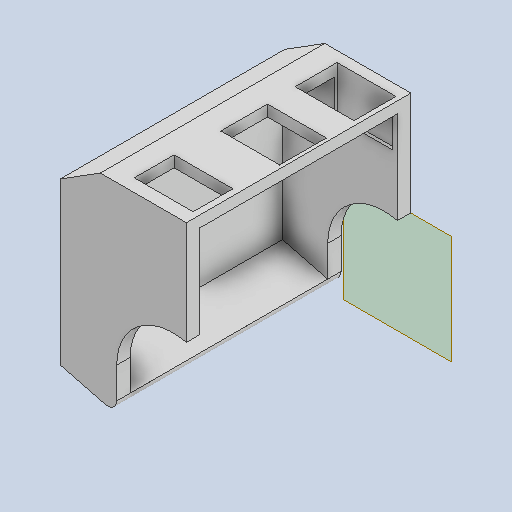
# Autodesk Inventor part: obudowa
Saved by Autodesk Inventor 2022 (Build 260153000, 153)
## iProperties
Created: 2022-12-13
Part Number: obudowa
Material: Generic
Document SubType Name: Modeling
Designer: komputer
Density: 1 g/cm^3
Appearance: Default
Author: komputer
Autodesk Inventor part; units mm, degrees
ref_plane "YZ Plane" through (0, 0, 0) normal (1, 0, 0) x (0, 1, 0)
ref_plane "XZ Plane" through (0, 0, 0) normal (0, 1, 0) x (-1, 0, 0)
ref_plane "XY Plane" through (0, 0, 0) normal (0, 0, 1) x (1, 0, 0)
sketch "Sketch1" plane through (0, 0, 0) normal (0, 0, 1) x (1, 0, 0)
  circle A0 centre (0, 0) radius 11 projected
  line L0 (9.8023, 37.5977) -> (3, 35.24) projected
  line L1 (3, 35.24) -> (3, 11.34) projected
  line L2 (3, 11.34) -> (9, 11.34) projected
  line L3 (9, 11.34) -> (9, 30.1331) projected
  line L4 (9, 30.1331) -> (7.9327, 24.5668) projected
  line L5 (7.9327, 24.5668) -> (7.3445, 24.6796) projected
  line L6 (7.3445, 24.6796) -> (9.8023, 37.5977) projected
  circle A1 centre (0, 0) radius 12.5167
  line L7 (-21, 24.5198) -> (-21, -3.96) projected
  line L8 (-19, -3.96) -> (-21, -3.96) projected
  line L9 (-19, 24.5198) -> (-19, -3.96) projected
  line L10 (-21, 24.5198) -> (-19, 24.5198) projected
  line L11 (-21, 28.5732) -> (-21, 24.5198) projected
  line L12 (-21, 24.5198) -> (-19, 24.5198) projected
  line L13 (-19, 28.5732) -> (-19, 24.5198) projected
  line L14 (-21, 28.5732) -> (-19, 28.5732) projected
  line L15 (1.6453, 33.2633) -> (-11.4547, 33.2633) projected
  line L16 (-19, 0.49) -> (-19, -3.96) projected
  line L17 (-14, 0.49) -> (-19, 0.49) projected
  line L18 (-14, -0.96) -> (-14, 0.49) projected
  arc A2 (-14, -0.96) -> (-11, -3.96) centre (-11, -0.96) ccw projected
  line L19 (-11, -3.96) -> (-19, -3.96) projected
  line L20 (3, 35.24) -> (-21, 35.24)
  line L21 (-11.4547, 35.24) -> (-22.0722, 28.5732)
  line L22 (-22.0722, 28.5732) -> (-23.4016, 30.6904)
  line L23 (-23.4016, 30.6904) -> (-12.7841, 37.3572)
  line L24 (-23.4016, 30.6904) -> (-25.0875, 29.6318)
  line L25 (-25.0875, 29.6318) -> (-25.0875, -6.2453)
  line L26 (-25.0875, -6.2453) -> (-5.3307, -11.3248)
  point P0 (0, 0)
  point P1 (3, 12.1518)
  point P2 (-16.156, 35.24)
  dimension "d0" = 2.5
  constraints: 14 end point, 2 point on line, 1 coincident, 1 horizontal, 1 parallel, 1 perpendicular, 1 vertical, 3 other
  measures "d0" distance of L21.end L22.end
extrude "Extrusion1" add sketch "Sketch1" against normal blind 3 contours L1 A1 A2 L18 L17 L9 L13 L14 L11 L7 L8 L19 L26 L25 L24 L22 L21 L20 | L21 L22 L23 L20 | A1 L19 L9 L17 L18 A2 | L8 L7 L10 L9 | L11 L14 L13 L10
ref_plane "Work Plane1" through (0, 0, -50) normal (0, 0, -1) x (1, 0, 0)
sketch "Sketch2" plane through (0, 0, -50) normal (0, 0, -1) x (1, 0, 0)
  line L0 (3, -35.24) -> (3, -12.1518) projected
  arc A0 (-5.3307, 11.3248) -> (3, -12.1518) centre (0, 0) ccw projected
  line L1 (-5.3307, 11.3248) -> (-25.0875, 6.2453) projected
  line L2 (-25.0875, 6.2453) -> (-25.0875, -29.6318) projected
  line L3 (-25.0875, -29.6318) -> (-16.156, -35.24) projected
  line L4 (-16.156, -35.24) -> (3, -35.24) projected
  point P0 (0, 0)
extrude "Extrusion2" add sketch "Sketch2" against normal blind 3
sketch "Sketch3" plane through (0, 0, -47) normal (0, 0, 1) x (1, 0, 0)
  line L0 (-25.0875, 29.6318) -> (-25.0875, -6.2453) projected
  line L1 (-25.0875, -6.2453) -> (-5.3307, -11.3248) projected
  arc A0 (3, 12.1518) -> (-5.3307, -11.3248) centre (0, 0) ccw projected
  line L2 (3, 12.1518) -> (3, 35.24) projected
  line L3 (3, 35.24) -> (-16.156, 35.24) projected
  line L4 (-16.156, 35.24) -> (-25.0875, 29.6318) projected
  line L5 (-25.0875, 29.6318) -> (-25.0875, -6.2453) projected
  line L6 (-25.0875, -6.2453) -> (-22.5875, -6.2453)
  line L7 (-22.5875, -6.2453) -> (-22.5875, 29.6318)
  line L8 (-22.5875, 29.6318) -> (-25.0875, 29.6318)
  line L9 (-25.0875, 29.6318) -> (-25.0875, -6.2453)
  line L10 (-16.156, 35.24) -> (-25.0875, 29.6318) projected
  line L11 (-20.6218, 32.4359) -> (-19.2923, 30.3187)
  line L12 (-19.2923, 30.3187) -> (-10.0223, 36.1394)
  line L13 (-10.0223, 36.1394) -> (-28.1615, 24.7497)
  line L14 (3, 12.1518) -> (3, 35.24) projected
  line L15 (3, 35.24) -> (-20.6218, 35.24)
  line L16 (-20.6218, 35.24) -> (-20.6218, 32.74)
  line L17 (-20.6218, 32.74) -> (3, 32.74)
  line L18 (3, 32.74) -> (3, 35.24)
  line L19 (-25.0875, -6.2453) -> (-5.3307, -11.3248) projected
  line L20 (-15.2091, -8.7851) -> (-14.5866, -6.3638)
  line L21 (-14.5866, -6.3638) -> (-34.8376, -1.1573)
  line L22 (-14.5866, -6.3638) -> (7.6026, -12.0686)
  point P0 (0, 0)
  point P1 (-9.9857, -7.5467)
  point P2 (-22.5875, -4.3067)
  point P3 (-22.5875, 28.2496)
  point P4 (-15.4362, 32.74)
  point P5 (3, 32.74)
  dimension "d5" = 2.5
  dimension "d6" = 2.5
  dimension "d7" = 2.5
  dimension "d8" = 2.5
  constraints: 28 end point, 6 parallel, 4 perpendicular, 2 horizontal, 2 midpoint, 1 collinear, 1 point on line
  measures "d5" distance of L8.end L7.end
  measures "d6" distance of L11.start L11.end
  measures "d7" distance of L16.end L15.end
  measures "d8" distance of L20.start L20.end
extrude "Extrusion3" add sketch "Sketch3" along normal up to surface (44 mm away) contours L8 L7 L13 L0 | L4 L11 L13 L7 L8 | L13 L7 L21 L0 | L4 L17 L12 L11 | L21 L7 L6 L0 | L4 L3 L12 L17 | L6 L7 L21 L20 L1 | L12 L3 L2 L17 | L20 L22 A0 L1
sketch "Sketch4" plane through (-16.156, 35.24, 0) normal (0, 1, 0) x (1, 0, 0)
  line L0 (19.156, 0) -> (0, 0) projected
  line L1 (19.156, 0) -> (19.156, 50) projected
  line L2 (0, 50) -> (19.156, 50) projected
  line L3 (0, 0) -> (0, 50) projected
  line L4 (18.4023, 21.528) -> (18.4023, 31.928) projected
  line L5 (5.3023, 21.528) -> (18.4023, 21.528) projected
  line L6 (5.3023, 31.928) -> (5.3023, 21.528) projected
  line L7 (18.4023, 31.928) -> (5.3023, 31.928) projected
  line L8 (5.039, 38.3353) -> (18.139, 38.3353) projected
  line L9 (18.139, 38.3353) -> (18.139, 47.6905) projected
  line L10 (5.039, 38.3353) -> (18.139, 38.3353) projected
  line L11 (18.139, 38.3353) -> (18.139, 47.6905) projected
  line L12 (5.039, 38.3353) -> (18.139, 38.3353) projected
  line L13 (5.039, 47.6905) -> (5.039, 38.3353) projected
  line L14 (18.139, 47.6905) -> (5.039, 47.6905) projected
  line L15 (17.8013, 2.855) -> (17.8013, 11.7262) projected
  line L16 (4.7013, 2.855) -> (17.8013, 2.855) projected
  line L17 (4.7013, 11.7262) -> (4.7013, 2.855) projected
  line L18 (17.8013, 11.7262) -> (4.7013, 11.7262) projected
  line L19 (18.4023, 21.528) -> (18.4023, 31.928) projected
  line L20 (5.3023, 21.528) -> (18.4023, 21.528) projected
  line L21 (5.3023, 31.928) -> (5.3023, 21.528) projected
  line L22 (18.4023, 31.928) -> (5.3023, 31.928) projected
  line L23 (5.039, 39.2089) -> (18.139, 39.2089) projected
  line L24 (18.139, 39.2089) -> (18.139, 48.5642) projected
  line L25 (17.8013, 1.8112) -> (17.8013, 10.6824) projected
  line L26 (17.8013, 11.7262) -> (17.8013, 10.6824) projected
  line L27 (17.8013, 11.7262) -> (4.7013, 11.7262) projected
  line L28 (17.8013, 1.8112) -> (17.8013, 10.6824) projected
  line L29 (17.8013, 2.855) -> (17.8013, 1.8112) projected
  point P0 (16.156, 0)
extrude "Extrusion4" cut sketch "Sketch4" against normal blind 10 contours L5 L6 L7 L4 | L13 L23 L9 L8 | L13 L14 L9 L23 | L16 L17 L18 L15
sketch "Sketch5" plane through (0, 0, -50) normal (0, 0, -1) x (-1, 0, 0)
  line L0 (25.0875, -6.2453) -> (25.0875, 29.6318) projected
  line L1 (25.0875, 29.6318) -> (16.156, 35.24) projected
  line L2 (16.156, 35.24) -> (-3, 35.24) projected
  line L3 (-3, 35.24) -> (-3, 12.1518) projected
  arc A0 (5.3307, -11.3248) -> (-3, 12.1518) centre (0, 0) ccw projected
  line L4 (5.3307, -11.3248) -> (25.0875, -6.2453) projected
  arc A1 (9.9857, -7.5467) -> (-3, 12.1518) centre (0, 0) ccw projected
  line L5 (12.5167, 0) -> (12.5167, -6.898)
  line L6 (25.0875, -6.2453) -> (15.0147, -8.835)
  line L7 (5.3307, -11.3248) -> (25.0875, -6.2453) projected
  arc A2 (12.5167, -6.898) -> (15.0147, -8.835) centre (14.5167, -6.898) ccw
  point P0 (0, 0)
  point P1 (12.5167, -9.4773)
  point P2 (15.0147, -8.835)
  point P3 (12.5167, 0)
  dimension "d13" = 2
  constraints: 4 end point, 3 point on circle, 3 point on line, 3 tangent, 1 centre point, 1 vertical
  measures "d13" radius of A2
extrude "Extrusion5" cut sketch "Sketch5" against normal through all contours L4 A0 L5 A2
body "Solid1"
